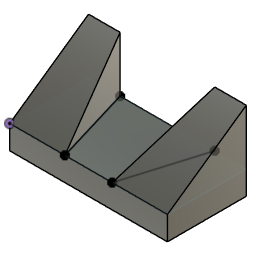
que3 v2 (Autodesk Fusion 360 design; units mm, degrees)
Autodesk Fusion 360 part; units mm, degrees
sketch "Sketch1" plane through (0, 0, 0) normal (0, 0, 1) x (1, 0, 0)
  line L0 (0, 0) -> (100, 0)
  line L1 (0, 0) -> (0, 50)
  line L2 (0, 50) -> (100, 50)
  line L3 (100, 50) -> (100, 0)
  dimension "d1" = 100
  dimension "d2" = 50
  constraint coincident L0.start L1.start
  constraint horizontal L0
  constraint perpendicular L0 L1
  constraint perpendicular L1 L2
  constraint perpendicular L0 L3
  measures "d1" distance of L0.start L0.end
  measures "d2" distance of L0.start L1.end
extrude "Extrude1" add sketch "Sketch1" along normal blind 15
sketch "Sketch2" plane through (0, 0, 15) normal (0, 0, 1) x (-1, 0, 0)
  line L0 (0, 0) -> (-100, 0)
  line L1 (-100, 0) -> (-100, -50)
  line L2 (-100, -50) -> (0, -50)
  line L3 (0, -50) -> (0, 0)
  line L4 (-20, -50) -> (-35, 0)
  line L5 (-80, -50) -> (-65, 0)
  dimension "d6" = 35
  dimension "d7" = 20
  dimension "d8" = 35
  dimension "d9" = 20
  constraint coincident L2 L4.start
  constraint coincident L0 L4.end
  constraint coincident L2 L5.start
  constraint coincident L0 L5.end
  measures "d6" distance of L0.start L4.end
  measures "d7" distance of L1.end L5.start
  measures "d8" distance of L0.end L5.end
  measures "d9" distance of L2.end L4.start
extrude "Extrude2" add sketch "Sketch2" along normal blind 35 contours L0 L2 L3 L4
extrude "Extrude3" add sketch "Sketch2" along normal blind 35 contours L0 L1 L2 L5
chamfer "Chamfer1" distance 50 distance2 35 1 edges at (17.5, 0, 50) measured on face at (18.3333, 16.6667, 50)
chamfer "Chamfer1" distance 50 distance2 35 1 edges at (82.5, 0, 50) measured on face at (81.6667, 16.6667, 50)
